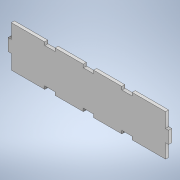
# Autodesk Inventor part: Стекнка t3
Saved by Autodesk Inventor 2021 (Build 250183000, 183)
## iProperties
Created: 2021-04-10
Part Number: Стекнка t3
Material: Типовые
Document SubType Name: Modeling
Designer: user
Density: 1 g/cm^3
Appearance: По умолчанию
Author: user
Autodesk Inventor part; units mm, degrees
ref_plane "YZ Plane" through (0, 0, 0) normal (1, 0, 0) x (0, 1, 0)
ref_plane "XZ Plane" through (0, 0, 0) normal (0, 1, 0) x (-1, 0, 0)
ref_plane "XY Plane" through (0, 0, 0) normal (0, 0, 1) x (1, 0, 0)
sketch "Эскиз1" plane through (0, 0, 0) normal (0, 0, 1) x (1, 0, 0)
  line L0 (-74.9994, 20) -> (-42.5, 20)
  line L1 (-42.5, 17) -> (-42.5, 20)
  line L2 (-42.5, -17) -> (-42.5, -20)
  line L3 (-74.9994, -20) -> (-42.5, -20)
  line L4 (-74.9994, -20) -> (-42.5, -20)
  line L5 (-74.9994, -5.9498) -> (-77.9994, -5.9498)
  line L6 (-74.9994, 20) -> (-42.5, 20)
  line L7 (-74.9994, 6.0502) -> (-77.9994, 6.0502)
  line L8 (32.5, 20) -> (32.5, 17)
  line L9 (32.5, -20) -> (5, -20)
  line L10 (32.5, -20) -> (5, -20)
  line L11 (5, 17) -> (5, 20)
  line L12 (32.5, 20) -> (5, 20)
  line L13 (0, 17) -> (5, 17)
  line L14 (32.5, 20) -> (5, 20)
  line L15 (75.0067, 20) -> (42.5, 20)
  line L16 (42.5, 17) -> (42.5, 20)
  line L17 (32.5, 17) -> (42.5, 17)
  line L18 (32.5, -20) -> (32.5, -17)
  line L19 (32.5, -17) -> (42.5, -17)
  line L20 (42.5, -17) -> (42.5, -20)
  line L21 (75.0067, 20) -> (42.5, 20)
  line L22 (75.0067, 5.8458) -> (78.0067, 5.8458)
  line L23 (75.0067, -6.1542) -> (78.0067, -6.1542)
  line L24 (75.0067, -20) -> (42.5, -20)
  line L25 (75.0067, -20) -> (42.5, -20)
  line L26 (-32.5, 20) -> (-32.5, 17)
  line L27 (-32.5, 17) -> (-42.5, 17)
  line L28 (-32.5, 20) -> (-5, 20)
  line L29 (0, 17) -> (-5, 17)
  line L30 (-5, 17) -> (-5, 20)
  line L31 (-32.5, -20) -> (-32.5, -17)
  line L32 (-32.5, 20) -> (-5, 20)
  line L33 (-5, -17) -> (-5, -20)
  line L34 (-32.5, -20) -> (-5, -20)
  line L35 (-32.5, -20) -> (-5, -20)
  line L36 (0, -17) -> (-5, -17)
  line L37 (0, -17) -> (5, -17)
  line L38 (5, -17) -> (5, -20)
  line L39 (-32.5, -17) -> (-42.5, -17)
  line L40 (-74.9994, 6.0502) -> (-74.9994, 20)
  line L41 (-74.9994, -5.9498) -> (-74.9994, -20)
  line L42 (-74.9994, 6.0502) -> (-77.9994, 6.0502)
  line L43 (-77.9994, 6.0502) -> (-77.9994, -5.9498)
  line L44 (-77.9994, -5.9498) -> (-74.9994, -5.9498)
  line L45 (75.0067, 20) -> (75.0067, 5.8458)
  line L46 (75.0067, -6.1542) -> (75.0067, -20)
  line L47 (75.0067, 5.8458) -> (78.0067, 5.8458)
  line L48 (78.0067, 5.8458) -> (78.0067, -6.1542)
  line L49 (78.0067, -6.1542) -> (75.0067, -6.1542)
  point P0 (0, 0)
  point P1 (0, 0)
  point P2 (0, 0)
  constraints: 100 end point, 4 horizontal, 3 parallel, 3 perpendicular, 2 point on line, 1 coincident
extrude "Выдавливание1" add sketch "Эскиз1" along normal blind 3
